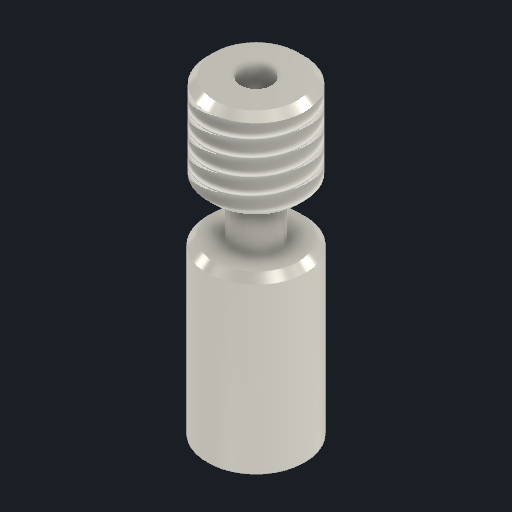
# Autodesk Inventor part: heatbreak ender 3s1
Saved by Autodesk Inventor 2024.3 (Build 283343000, 343)
## iProperties
Created: 2024-03-20
Part Number: heatbreak ender 3s1
Material: Titanium
Document SubType Name: Modeling
Designer: mateu
Appearance: Titanium
Surface Area: 5.15948 cm^2
Volume: 0.403862 cm^3
Author: mateu
Autodesk Inventor part; units mm, degrees
ref_plane "YZ Plane" through (0, 0, 0) normal (1, 0, 0) x (0, 1, 0)
ref_plane "XZ Plane" through (0, 0, 0) normal (0, 1, 0) x (-1, 0, 0)
ref_plane "XY Plane" through (0, 0, 0) normal (0, 0, 1) x (1, 0, 0)
sketch "Sketch1" plane through (0, 0, 0) normal (0, 0, 1) x (1, 0, 0)
  line L0 (0, 0) -> (2.9, 0)
  line L1 (3, 0.1) -> (3, 10.5)
  line L2 (3, 10.5) -> (1.35, 10.5)
  line L3 (1.35, 10.5) -> (1.35, 13.5)
  line L4 (1.35, 13.5) -> (2.95, 13.5)
  line L5 (2.95, 13.5) -> (2.95, 19)
  line L6 (2.95, 19) -> (0.95, 19)
  line L7 (0.95, 19) -> (0.95, 0)
  line L8 (2.9, 0) -> (3, 0.1)
  line L9 (0.95, 0) -> (1.95, 0)
  line L10 (1.95, 0) -> (0.95, 0.5774)
  line L11 (0, 17.1506) -> (0, 0) construction
  dimension "d15" = 2.9
  dimension "d16" = 10.4
  dimension "d17" = 1.65
  dimension "d18" = 1.6
  dimension "d19" = 5.5
  dimension "d20" = 90
  dimension "d21" = 2
  dimension "d22" = 90
  dimension "d23" = 1
  dimension "d24" = 30
  dimension "d25" = 19
  constraints: 24 end point, 7 perpendicular, 3 point on line, 1 horizontal, 1 vertical
  measures "d15" distance of L0.start L0.end
  measures "d16" distance of L1.start L1.end
  measures "d17" distance of L1.end L2.end
  measures "d18" distance of L3.end L4.end
  measures "d19" distance of L4.end L5.end
  measures "d20" angle of L5 L4
  measures "d21" distance of L5.end L6.end
  measures "d22" angle of L6 L5
  measures "d23" distance of L7.end L9.end
  measures "d24" angle of L10 L9
  measures "d25" distance between parallel lines of L0 L6
revolve "Revolution1" add sketch "Sketch1" angle 360 about axis through (0, 17.1506, 0) along (0, -1, 0) contours L10 L7 L6 L5 L4 L3 L2 L1 L8 L0
thread "Thread1" size "M6x1" class "6g" standard "ANSI Metric M Profile" length 5.3
chamfer "Chamfer1" distance 0.4 angle 45 2 edges at (-2.95, 19, 0) (-2.95, 13.5, 0)
chamfer "Chamfer2" distance 0.4 angle 45 1 edges at (-3, 10.5, 0)
body "Solid1"
